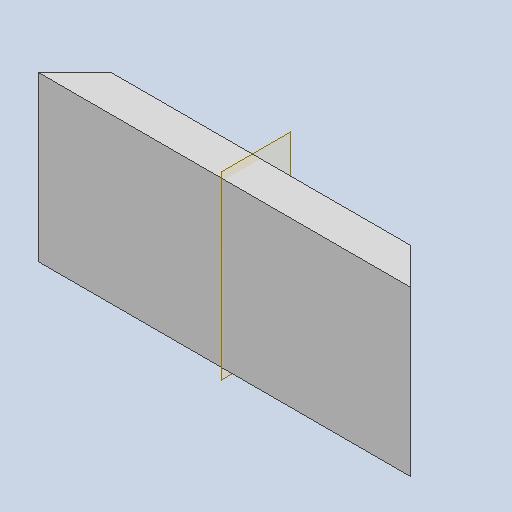
# Autodesk Inventor part: PDMS Chamber-Mold-V8-Top_Bottom-Wall Steven
Saved by Autodesk Inventor 2022 (Build 260153000, 153)
## iProperties
Created: 2021-11-29
Part Number: PDMS Chamber-Mold-V8-Top_Bottom-Wall Steven
Material: Generic
Document SubType Name: Modeling
Designer: Hirota Lab
Density: 1 g/cm^3
Appearance: Default
Author: Hirota Lab
Autodesk Inventor part; units mm, degrees
ref_plane "XZ Plane" through (0, 0, 0) normal (0, 1, 0) x (-1, 0, 0)
ref_plane "XY Plane" through (0, 0, 0) normal (0, 0, 1) x (1, 0, 0)
sketch "Sketch1" plane through (0, 0, 0) normal (0, 1, 0) x (-1, 0, 0)
  line L0 (0, 0) -> (41, 0)
  line L1 (0, 0) -> (41, 0) construction
  line L2 (4, -4) -> (37, -4)
  line L3 (0, -4) -> (37, -4) construction
  line L4 (37, -4) -> (41, 0)
  line L5 (0, 0) -> (4, -4)
  dimension "d0" = 41
  dimension "d1" = 0
  dimension "d4" = 0
  constraints: 12 end point, 4 horizontal, 1 collinear, 1 perpendicular
  measures "d0" distance of L0.start L0.end
  measures "d1" distance between parallel lines of L0 L1
  measures "d4" distance between parallel lines of L2 L3
extrude "Extrusion1" add sketch "Sketch1" along normal blind 18.05
sketch "Sketch2" plane through (-4, 0, -4) normal (0, 0, -1) x (-1, 0, 0)
  line L0 (-4, 0) -> (-4, 18.05) projected
  line L1 (37, 0) -> (37, 18.05) projected
  line L2 (-4, 6.1) -> (37, 6.1)
  line L3 (37, 6.1) -> (37, 2)
  line L4 (37, 2) -> (-4, 2)
  line L5 (-4, 2) -> (-4, 6.1)
  line L6 (0, 0) -> (33, 0) projected
  point P0 (-4, 2)
  dimension "d7" = 4.1
  dimension "d8" = 2
  constraints: 8 end point, 2 parallel, 2 point on line, 1 horizontal, 1 perpendicular
  measures "d7" distance of L2.end L3.end
  measures "d8" distance between parallel lines of L6 L4
extrude "Extrusion2" cut sketch "Sketch2" against normal blind 2
ref_plane "Work Plane1" through (-20.5, 0, 0) normal (1, 0, 0) x (0, 1, 0)
body "Solid1"
